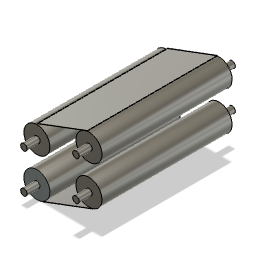
paper tensioning mechanism v1 (Autodesk Fusion 360 design; units mm, degrees)
Autodesk Fusion 360 part; units mm, degrees
sketch "Sketch1" plane through (0, 0, 0) normal (0, 0, 1) x (1, 0, 0)
  circle A0 centre (0, 0) radius 50
  dimension "d1" = 100
  constraint coincident A0.centre origin
  measures "d1" diameter of A0
extrude "Extrude1" add sketch "Sketch1" along normal blind 500 makes body 1
sketch "Sketch2" plane through (0, 0, 500) normal (0, 0, 1) x (1, 0, 0)
  circle A0 centre (0, 0) radius 50
  circle A1 centre (0, 0) radius 12.5
  dimension "d4" = 25
  constraint coincident A0.centre A1.centre
  measures "d4" diameter of A1
extrude "Extrude2" add sketch "Sketch2" along normal blind 50 contours A1 bodies 1
sketch "Sketch3" plane through (0, 0, 0) normal (0, 0, 1) x (1, 0, 0)
  circle A0 centre (0, 0) radius 12.5
  dimension "d7" = 25
  constraint coincident A0.centre origin
  measures "d7" diameter of A0
extrude "Extrude3" add sketch "Sketch3" against normal blind 50 bodies 1
copy_body "CopyPasteBodies1" bodies 1 makes body 2
move_body "Move1" bodies 2 to x (1, 0, 0) y (0, 1, 0) z (0, 0, 1) at (200, 0, 0)
move_body "Move2" bodies 2 to x (1, 0, 0) y (0, 1, 0) z (0, 0, 1) at (0, 75, 0)
copy_body "CopyPasteBodies2" bodies 1 makes body 3
move_body "Move3" bodies 3 to x (1, 0, 0) y (0, 1, 0) z (0, 0, 1) at (0, 150, 0)
copy_body "CopyPasteBodies3" bodies 2 makes body 4
move_body "Move4" bodies 4 to x (1, 0, 0) y (0, 1, 0) z (0, 0, 1) at (0, 150, 0)
sketch "Sketch4" plane through (0, 0, 500) normal (0, 0, 1) x (1, 0, 0)
  circle A0 centre (0, 0) radius 12.5
  circle A1 centre (0, 0) radius 50
sketch "Sketch5" plane through (0, 0, 0) normal (0, 0, 1) x (1, 0, 0)
sketch "Sketch6" plane through (0, 0, 0) normal (0, 0, 1) x (1, 0, 0)
sketch "Sketch7" plane through (0, 0, 0) normal (0, 0, 1) x (1, 0, 0)
  line L0 (22, -45) -> (214, 27)
  line L1 (214, 27) -> (214.3511, 26.0637)
  line L2 (22, -45) -> (22.3511, -45.9363)
  line L3 (22.3511, -45.9363) -> (214.3511, 26.0637)
  dimension "d11" = 1
  dimension "d12" = 1
  constraint perpendicular L0 L1
  constraint perpendicular L0 L2
  measures "d11" distance of L0.end L1.end
  measures "d12" distance of L0.start L2.end
extrude "Extrude4" add sketch "Sketch7" along normal blind 500 separate body makes body 5
copy_body "CopyPasteBodies4" bodies 5 makes body 6
move_body "Move5" bodies 6 to x (1, 0, 0) y (0, 1, 0) z (0, 0, 1) at (-20, 250, 0)
named bodies: "guide roller", "guide roller (1)", "guide roller (1) (1)", "guide roller (1) (1) (1)"
